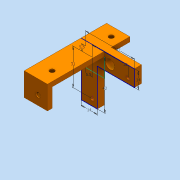
# Autodesk Inventor part: MotorMountRight
Saved by Autodesk Inventor 2016 (Build 200138000, 138)
## iProperties
Created: 2016-08-20
Part Number: MotorMountRight
Material: PLA Orange
Document SubType Name: Modeling
Designer: Sam
Density: 1 g/cm^3
Appearance: Generic
Author: Sam
Autodesk Inventor part; units mm, degrees
ref_plane "YZ Plane" through (0, 0, 0) normal (1, 0, 0) x (0, 1, 0)
ref_plane "XZ Plane" through (0, 0, 0) normal (0, 1, 0) x (-1, 0, 0)
ref_plane "XY Plane" through (0, 0, 0) normal (0, 0, 1) x (1, 0, 0)
sketch "Sketch1" plane through (0, 0, 0) normal (0, 1, 0) x (-1, 0, 0)
  line L0 (0, 0) -> (-20, 0)
  line L1 (-20, 0) -> (-20, -20)
  line L2 (-20, -20) -> (0, -20)
  line L3 (0, -20) -> (0, 0)
  dimension "d0" = 20
  dimension "d1" = 20
  constraints: 8 end point, 2 parallel, 1 horizontal, 1 perpendicular
  measures "d0" distance of L2.end L1.end
  measures "d1" distance of L1.end L0.end
extrude "Extrusion1" add sketch "Sketch1" along normal blind 4
sketch "Sketch2" plane through (0, 4, 0) normal (0, 1, 0) x (1, 0, 0)
  line L0 (0, 0) -> (20, 0)
  line L1 (20, 0) -> (20, 4)
  line L2 (20, 4) -> (4, 4)
  line L3 (0, 4) -> (0, 0)
  line L4 (0, 0) -> (4, 0)
  line L5 (4, 20) -> (0, 20)
  line L6 (0, 20) -> (0, 0)
  line L7 (4, 4) -> (4, 20)
  line L8 (0, 0) -> (20, 0) projected
  line L9 (0, 0) -> (20, 0)
  line L10 (0, 20) -> (0, 0) projected
  line L11 (0, 0) -> (0, 20)
  constraints: 20 end point, 4 parallel, 3 horizontal, 2 perpendicular, 1 vertical
extrude "Extrusion2" add sketch "Sketch2" along normal blind 45
hole "Hole2" at (12, 12, -4) direction (0, 0, 1) diameter 4 end through all
hole "Hole3" at (4, 12, -12) direction (-1, 0, 0) diameter 4 end through all
hole "Hole4" at (12, 4, -12) direction (0, -1, 0) diameter 4 end through all
sketch "Sketch3" plane through (20, 4, -4) normal (0, 0, -1) x (-1, 0, 0)
  line L0 (12.0415, 8) -> (10.0207, 4.5)
  line L1 (10.0207, 4.5) -> (5.9793, 4.5)
  line L2 (5.9793, 4.5) -> (3.9585, 8)
  line L3 (3.9585, 8) -> (5.9793, 11.5)
  line L4 (5.9793, 11.5) -> (10.0207, 11.5)
  line L5 (10.0207, 11.5) -> (12.0415, 8)
  point P0 (20, -4)
  point P1 (8, 8)
  dimension "d51" = 7
  constraints: 12 end point, 13 other
  measures "d51" distance between parallel lines of L4 L1
sketch "Sketch4" plane through (4, 4, -4) normal (1, 0, 0) x (0, 0, -1)
  line L0 (12.0415, 8) -> (10.0207, 4.5)
  line L1 (10.0207, 4.5) -> (5.9793, 4.5)
  line L2 (5.9793, 4.5) -> (3.9585, 8)
  line L3 (3.9585, 8) -> (5.9793, 11.5)
  line L4 (5.9793, 11.5) -> (10.0207, 11.5)
  line L5 (10.0207, 11.5) -> (12.0415, 8)
  point P0 (-4, -4)
  point P1 (8, 8)
  dimension "d52" = 7
  constraints: 12 end point, 13 other
  measures "d52" distance between parallel lines of L4 L1
sketch "Sketch5" plane through (0, 4, 0) normal (0, 1, 0) x (1, 0, 0)
  circle A0 centre (12, 12) radius 2 projected
  line L0 (12, 7.9585) -> (8.5, 9.9793)
  line L1 (8.5, 9.9793) -> (8.5, 14.0207)
  line L2 (8.5, 14.0207) -> (12, 16.0415)
  line L3 (12, 16.0415) -> (15.5, 14.0207)
  line L4 (15.5, 14.0207) -> (15.5, 9.9793)
  line L5 (15.5, 9.9793) -> (12, 7.9585)
  point P0 (0, 0)
  dimension "d53" = 7
  constraints: 12 end point, 1 coincident, 13 other
  measures "d53" distance between parallel lines of L1 L4
extrude "Extrusion3" cut sketch "Sketch3" against normal blind 3.2
extrude "Extrusion4" cut sketch "Sketch4" against normal blind 3.2
extrude "Extrusion5" cut sketch "Sketch5" against normal blind 3.2
sketch "Sketch6" plane through (0, 49, 0) normal (0, 1, 0) x (1, 0, 0)
  line L0 (0, 0) -> (20, 0) projected
  line L1 (0, 0) -> (0, 46)
  line L2 (0, 20) -> (0, 0) projected
  line L3 (0, 0) -> (46, 0)
  line L4 (46, 0) -> (46, 14)
  line L5 (0, 46) -> (14, 46)
  line L6 (14, 46) -> (14, 14)
  line L7 (14, 14) -> (46, 14)
  line L8 (20, 4) -> (4, 4) projected
  line L9 (4, 4) -> (4, 20) projected
  line L10 (20, 20) -> (4, 20) projected
  line L11 (20, 4) -> (20, 20) projected
  point P0 (9.5, 9.5)
  point P1 (9.5, 40.5)
  point P2 (40.5, 9.5)
  dimension "d62" = 14
  dimension "d65" = 42
  dimension "d66" = 42
  dimension "d68" = 5.5
  dimension "d69" = 5.5
  dimension "d70" = 31
  dimension "d71" = 31
  dimension "d72" = 14
  constraints: 12 end point, 3 perpendicular, 1 collinear, 1 horizontal, 1 point on line
  measures "d62" distance of L1.end L5.end
  measures "d65" distance between parallel lines of L5 L8
  measures "d66" distance between parallel lines of L4 L9
  measures "d68" distance from line of L9 point (9.5, 9.5)
  measures "d69" distance from line of L8 point (9.5, 9.5)
  measures "d70" distance of point (40.5, 9.5) point (9.5, 9.5)
  measures "d71" distance of point (9.5, 9.5) point (9.5, 40.5)
  measures "d72" distance of L3.end L4.end
extrude "Extrusion6" add sketch "Sketch6" along normal blind 6 contours L1 L5 L6 L10 L9 L8 L11 L7 L4 L3 L0 | L11 L8 L9 L10 L6 L7
hole "Hole5" at (9.5, 49, -9.5) at (9.5, 49, -40.5) at (40.5, 49, -9.5) direction (0, 1, 0) diameter 3 end through all
sketch "Sketch7" plane through (0, 55, 0) normal (0, 1, 0) x (1, 0, 0)
  line L0 (0, 0) -> (20, 0) projected
  line L1 (20, 4) -> (4, 4) projected
  line L2 (0, 0) -> (20, 0)
  line L3 (20, 0) -> (20, 4)
  line L4 (20, 4) -> (4, 4)
  line L5 (0, 4) -> (0, 0)
  line L6 (0, 0) -> (4, 0)
  line L7 (4, 20) -> (0, 20)
  line L8 (0, 20) -> (0, 0)
  line L9 (4, 4) -> (4, 20)
  dimension "d82" = 20
  dimension "d83" = 4
  dimension "d84" = 4
  dimension "d85" = 20
  constraints: 16 end point, 4 parallel, 2 horizontal, 2 perpendicular
  measures "d82" distance of L5.start L1.start
  measures "d83" distance of L1.start L2.end
  measures "d84" distance of L7.end L7.start
  measures "d85" distance of L7.start L6.end
extrude "Extrusion7" add sketch "Sketch7" along normal blind 16
hole "Hole6" at (12, 63, -4) direction (0, 0, 1) diameter 4 end through all
hole "Hole7" at (4, 63, -12) direction (-1, 0, 0) diameter 4 end through all
sketch "Sketch8" plane through (4, 55, -4) normal (1, 0, 0) x (0, 0, -1)
  line L0 (3.9585, 8) -> (5.9793, 11.5)
  line L1 (5.9793, 11.5) -> (10.0207, 11.5)
  line L2 (10.0207, 11.5) -> (12.0415, 8)
  line L3 (12.0415, 8) -> (10.0207, 4.5)
  line L4 (10.0207, 4.5) -> (5.9793, 4.5)
  line L5 (5.9793, 4.5) -> (3.9585, 8)
  point P0 (-4, -55)
  point P1 (8, 8)
  dimension "d106" = 7
  constraints: 12 end point, 13 other
  measures "d106" distance between parallel lines of L1 L4
sketch "Sketch9" plane through (20, 55, -4) normal (0, 0, -1) x (-1, 0, 0)
  circle A0 centre (8, 8) radius 2 projected
  line L0 (3.9585, 8) -> (5.9793, 11.5)
  line L1 (5.9793, 11.5) -> (10.0207, 11.5)
  line L2 (10.0207, 11.5) -> (12.0415, 8)
  line L3 (12.0415, 8) -> (10.0207, 4.5)
  line L4 (10.0207, 4.5) -> (5.9793, 4.5)
  line L5 (5.9793, 4.5) -> (3.9585, 8)
  point P0 (20, -55)
  dimension "d107" = 7
  constraints: 12 end point, 1 coincident, 13 other
  measures "d107" distance between parallel lines of L1 L4
extrude "Extrusion8" cut sketch "Sketch9" against normal blind 3.2
extrude "Extrusion9" cut sketch "Sketch8" against normal blind 3.2
hole "Hole8" at (25, 55, -7) direction (0, -1, 0) diameter 8 end through all
body "Solid1"
